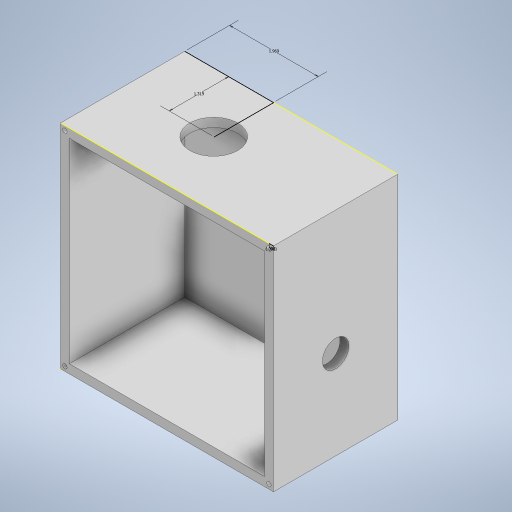
# Autodesk Inventor part: 3d_enclosure_2_19_1
Saved by Autodesk Inventor 2024 (Build 280153000, 153)
## iProperties
Created: 2024-02-19
Part Number: 3d_enclosure_2_19_1
Material: Generic
Document SubType Name: Modeling
Designer: jtw4137
Density: 1 g/cm^3
Appearance: Default
Author: jtw4137
Autodesk Inventor part; units mm, degrees
ref_plane "YZ Plane" through (0, 0, 0) normal (1, 0, 0) x (0, 1, 0)
ref_plane "XZ Plane" through (0, 0, 0) normal (0, 1, 0) x (-1, 0, 0)
ref_plane "XY Plane" through (0, 0, 0) normal (0, 0, 1) x (1, 0, 0)
sketch "Sketch18" plane through (0, 0, 0) normal (0, 0, 1) x (1, 0, 0)
  line L0 (0, 0) -> (120, 0)
  line L1 (120, 0) -> (120, 120)
  line L2 (120, 120) -> (0, 120)
  line L3 (0, 120) -> (0, 0)
  dimension "d90" = 120
  dimension "d91" = 120
  dimension "d92" = 120
  dimension "d93" = 120
  constraints: 8 end point, 2 perpendicular, 1 horizontal
  measures "d90" distance of L0.start L0.end
  measures "d91" distance of L0.end L1.end
  measures "d92" distance of L1.end L2.end
  measures "d93" distance of L2.end L0.start
extrude "Extrusion4" add sketch "Sketch18" along normal blind 70
sketch "Sketch20" plane through (0, 0, 70) normal (0, 0, 1) x (1, 0, 0)
  point P0 (0, 0)
sketch "Sketch21" plane through (0, 0, 70) normal (0, 0, 1) x (1, 0, 0)
  line L0 (120, 120) -> (0, 120) projected
  line L1 (0, 120) -> (0, 115)
  line L2 (0, 120) -> (0, 0) projected
  line L3 (0, 115) -> (115, 115)
  line L4 (115, 115) -> (115, 5)
  line L5 (115, 5) -> (5, 5)
  line L6 (5, 5) -> (5, 115)
  dimension "d102" = 5
  dimension "d103" = 115
  dimension "d104" = 110
  dimension "d105" = 110
  dimension "d106" = 110
  constraints: 10 end point, 2 perpendicular, 2 point on line, 1 horizontal
  measures "d102" distance of L0.end L1.end
  measures "d103" distance of L1.end L3.end
  measures "d104" distance of L3.end L4.end
  measures "d105" distance of L4.end L5.end
  measures "d106" distance of L5.end L6.end
sketch "Sketch23" plane through (0, 0, 70) normal (0, 0, 1) x (1, 0, 0)
  line L0 (5.0371, 115.0535) -> (115.0371, 115.0535)
  line L1 (115.0371, 115.0535) -> (115.0371, 5.0535)
  line L2 (115.0371, 5.0535) -> (5.0371, 5.0535)
  line L3 (5.0371, 5.0535) -> (5.0371, 115.0535)
  line L4 (0, 0) -> (2.5, 0)
  line L5 (0, 0) -> (120, 0) projected
  line L6 (2.5, 0) -> (2.5, 2.5)
  circle A0 centre (2.5, 2.5) radius 1.25
  dimension "d108" = 110
  dimension "d109" = 110
  dimension "d110" = 110
  dimension "d143" = 2.5
  dimension "d144" = 2.5
  dimension "d145" = 2.5
  constraints: 12 end point, 3 perpendicular, 1 centre point, 1 coincident, 1 horizontal, 1 point on line
  measures "d108" distance of L0.start L0.end
  measures "d109" distance of L0.end L1.end
  measures "d110" distance of L1.end L2.end
  measures "d143" distance of L4.start L4.end
  measures "d144" distance of L4.end L6.end
  measures "d145" diameter of A0
extrude "Extrusion5" cut sketch "Sketch21" against normal blind 65
sketch "Sketch24" plane through (5, 115, 70) normal (0, -1, 0) x (1, 0, 0)
  point P0 (-5, -70)
sketch "Sketch25" plane through (0, 120, 0) normal (0, 1, 0) x (1, 0, 0)
  line L0 (0, 0) -> (120, 0) projected
  line L1 (0, 0) -> (50, 0)
  line L2 (50, 0) -> (50, -33.5)
  dimension "d113" = 50
  dimension "d114" = 33.5
  constraints: 4 end point, 1 collinear, 1 perpendicular
  measures "d113" distance of L0.start L1.end
  measures "d114" distance of L1.end L2.end
sketch "Sketch26" plane through (0, 120, 0) normal (0, 1, 0) x (1, 0, 0)
  circle A0 centre (49.9198, -33.5778) radius 13.5
  point P0 (0, 0)
  dimension "d116" = 27
  constraints: 1 centre point
  measures "d116" diameter of A0
hole "Hole7" at (49.9198, 120, 33.5778) direction (0, -1, 0) diameter 27 depth 30
sketch "Sketch27" plane through (120, 0, 0) normal (1, 0, 0) x (0, 0, -1)
  line L0 (0, 0) -> (0, 50)
  line L1 (0, 120) -> (0, 0) projected
  line L2 (0, 50) -> (-35, 50)
  circle A0 centre (-35, 50) radius 7.5
  dimension "d124" = 50
  dimension "d125" = 35
  dimension "d126" = 15
  constraints: 4 end point, 1 centre point, 1 coincident, 1 horizontal, 1 point on line
  measures "d124" distance of L0.start L0.end
  measures "d125" distance of L0.end L2.end
  measures "d126" diameter of A0
hole "Hole8" at (120, 50, 35) direction (-1, 0, 0) diameter 15 depth 30
sketch "Sketch28" plane through (0, 0, 70) normal (0, 0, 1) x (1, 0, 0)
  line L0 (0, 120) -> (0, 0) projected
  line L1 (0, 120) -> (2.5, 120)
  line L2 (120, 120) -> (0, 120) projected
  line L3 (2.5, 120) -> (2.5, 117.5)
  dimension "d134" = 2.5
  dimension "d135" = 2.5
  constraints: 4 end point, 1 perpendicular, 1 point on line
  measures "d134" distance of L0.start L1.end
  measures "d135" distance of L1.end L3.end
hole "Hole9" at (2.5, 117.5, 70) direction (0, 0, -1) diameter 2.5 depth 38.1 tip angle 118
hole "Hole10" at (2.5, 2.5, 70) direction (0, 0, -1) diameter 2.5 depth 38.1 tip angle 118
sketch "Sketch29" plane through (115, 5, 70) normal (-1, 0, 0) x (0, 0, 1)
  point P0 (-70, -5)
sketch "Sketch30" plane through (0, 0, 70) normal (0, 0, 1) x (1, 0, 0)
  line L0 (120, 120) -> (0, 120) projected
  line L1 (120, 120) -> (117.5, 120)
  line L2 (117.5, 120) -> (120, 120)
  point P0 (0, 0)
  dimension "d153" = 2.5
  dimension "d154" = 2.5
  constraints: 4 end point, 1 collinear, 1 point on line
  measures "d153" distance of L0.start L1.end
  measures "d154" distance of L1.end L0.start
sketch "Sketch31" plane through (0, 0, 70) normal (0, 0, 1) x (1, 0, 0)
  line L0 (120, 120) -> (0, 120) projected
  line L1 (117.5038, 120) -> (120.0038, 120)
  line L2 (120.0038, 120) -> (120.0038, 117.5)
  line L3 (120.0038, 117.5) -> (117.5038, 117.5)
  point P0 (0, 0)
  dimension "d155" = 2.5
  dimension "d156" = 2.5
  dimension "d157" = 2.5
  constraints: 6 end point, 2 perpendicular, 1 collinear, 1 point on line
  measures "d155" distance of L1.start L1.end
  measures "d156" distance of L1.end L2.end
  measures "d157" distance of L2.end L3.end
hole "Hole11" at (117.5038, 117.5, 70) direction (0, 0, -1) diameter 2.5 depth 38.1 tip angle 118
sketch "Sketch32" plane through (0, 0, 70) normal (0, 0, 1) x (1, 0, 0)
  line L0 (0, 0) -> (120, 0) projected
  line L1 (120, 0) -> (120, 2.5)
  line L2 (120, 0) -> (120, 120) projected
  line L3 (120, 2.5) -> (117.5, 2.5)
  dimension "d165" = 2.5
  dimension "d166" = 2.5
  constraints: 4 end point, 1 perpendicular, 1 point on line
  measures "d165" distance of L0.end L1.end
  measures "d166" distance of L1.end L3.end
hole "Hole12" at (117.5, 2.5, 70) direction (0, 0, -1) diameter 2.5 depth 38.1 tip angle 118
body "Solid2"
